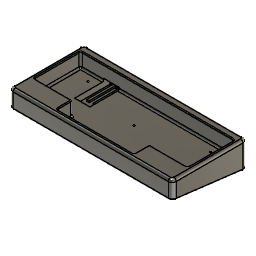
case-file (Autodesk Fusion 360 design; units mm, degrees)
Autodesk Fusion 360 part; units mm, degrees
sketch "Sketch1" plane through (0, 0, 0) normal (0, 0, 1) x (1, 0, 0)
  line L0 (0.9508, 78.7767) -> (191.4508, 78.7767)
  line L1 (0.4508, 79.2767) -> (191.9508, 79.2767)
  line L2 (60.6255, 57.2023) -> (74.6248, 57.2023)
  line L3 (79.6755, 57.2023) -> (93.6748, 57.2023)
  line L4 (0.9508, 89.2767) -> (191.4508, 89.2767)
  line L5 (60.6255, 76.2523) -> (74.6248, 76.2523)
  line L6 (55.5748, 62.253) -> (41.5755, 62.253)
  line L7 (79.6755, 24.1528) -> (79.6755, 38.1522)
  line L8 (60.6255, 24.1528) -> (60.6255, 38.1522)
  line L9 (41.5755, 57.2023) -> (55.5748, 57.2023)
  line L10 (55.5748, 57.2023) -> (55.5748, 43.203)
  line L11 (191.9508, 2.0769) -> (0.4508, 2.0769)
  line L12 (79.6755, 62.253) -> (79.6755, 76.2523)
  line L13 (136.8258, 62.253) -> (136.8258, 76.2523)
  line L14 (117.7738, 76.2523) -> (131.7748, 76.2523)
  line L15 (150.8248, 57.2023) -> (150.8248, 43.203)
  line L16 (131.7748, 24.1528) -> (117.7738, 24.1528)
  line L17 (74.6248, 76.2523) -> (74.6248, 62.253)
  line L18 (131.7748, 43.203) -> (117.7738, 43.203)
  line L19 (188.9248, 43.203) -> (174.9258, 43.203)
  line L20 (79.6755, 43.203) -> (79.6755, 57.2023)
  line L21 (3.4754, 62.253) -> (3.4754, 76.2523)
  line L22 (188.9248, 62.253) -> (174.9258, 62.253)
  line L23 (67.4811, 5.1029) -> (53.4818, 5.1029)
  line L24 (117.7738, 43.203) -> (117.7738, 57.2023)
  line L25 (112.7248, 24.1528) -> (98.7241, 24.1528)
  line L26 (131.7748, 57.2023) -> (131.7748, 43.203)
  line L27 (191.4508, 78.7767) -> (191.4508, 2.5769)
  line L28 (101.1068, 5.1029) -> (101.1068, 19.1023)
  line L29 (155.8758, 24.1528) -> (155.8758, 38.1522)
  line L30 (0.9508, 89.2767) -> (-5.5492, 89.2767)
  line L31 (155.8758, 62.253) -> (155.8758, 76.2523)
  line L32 (144.3188, 5.1029) -> (144.3188, 2.0769)
  line L33 (112.7248, 62.253) -> (98.7241, 62.253)
  line L34 (98.7241, 57.2023) -> (112.7248, 57.2023)
  line L35 (22.5255, 24.1528) -> (22.5255, 38.1522)
  line L36 (41.5755, 62.253) -> (41.5755, 76.2523)
  line L37 (136.8258, 43.203) -> (136.8258, 57.2023)
  line L38 (17.475, 43.203) -> (3.4754, 43.203)
  line L39 (115.1058, 19.1023) -> (115.1058, 5.1029)
  line L40 (188.9248, 57.2023) -> (188.9248, 43.203)
  line L41 (77.2929, 5.1029) -> (77.2929, 19.1023)
  line L42 (48.0818, 5.1029) -> (48.0818, 2.0769)
  line L43 (48.0818, 21.1278) -> (48.0818, 5.1029)
  line L44 (174.9258, 43.203) -> (174.9258, 57.2023)
  line L45 (155.8758, 43.203) -> (155.8758, 57.2023)
  line L46 (74.6248, 38.1522) -> (74.6248, 24.1528)
  line L47 (36.5248, 24.1528) -> (22.5255, 24.1528)
  line L48 (191.9508, 79.2767) -> (191.9508, 2.0769)
  line L49 (150.8248, 76.2523) -> (150.8248, 62.253)
  line L50 (36.5248, 43.203) -> (22.5255, 43.203)
  line L51 (169.8748, 24.1528) -> (155.8758, 24.1528)
  line L52 (143.8188, 5.1029) -> (143.8188, 2.0769)
  line L53 (3.4754, 24.1528) -> (3.4754, 38.1522)
  line L54 (115.1058, 5.1029) -> (101.1068, 5.1029)
  line L55 (138.9188, 5.1029) -> (124.9178, 5.1029)
  line L56 (197.9508, 85.2767) -> (197.9508, -3.9231)
  line L57 (188.9248, 76.2523) -> (188.9248, 62.253)
  line L58 (188.9248, 38.1522) -> (188.9248, 24.1528)
  line L59 (188.9248, 24.1528) -> (174.9258, 24.1528)
  line L60 (112.7248, 76.2523) -> (112.7248, 62.253)
  line L61 (101.1068, 19.1023) -> (115.1058, 19.1023)
  line L62 (169.8748, 43.203) -> (155.8758, 43.203)
  line L63 (48.5818, 21.6278) -> (48.5818, 5.1029)
  line L64 (17.475, 24.1528) -> (3.4754, 24.1528)
  line L65 (77.2929, 19.1023) -> (91.2936, 19.1023)
  line L66 (144.3188, 21.1278) -> (144.3188, 5.1029)
  line L67 (22.5255, 57.2023) -> (36.5248, 57.2023)
  line L68 (174.9258, 24.1528) -> (174.9258, 38.1522)
  line L69 (60.6255, 43.203) -> (60.6255, 57.2023)
  line L70 (174.9258, 57.2023) -> (188.9248, 57.2023)
  line L71 (3.4754, 57.2023) -> (17.475, 57.2023)
  line L72 (79.6755, 76.2523) -> (93.6748, 76.2523)
  line L73 (3.4754, 21.1278) -> (48.0818, 21.1278)
  line L74 (60.6255, 62.253) -> (60.6255, 76.2523)
  line L75 (136.8258, 24.1528) -> (136.8258, 38.1522)
  line L76 (174.9258, 62.253) -> (174.9258, 76.2523)
  line L77 (91.2936, 5.1029) -> (77.2929, 5.1029)
  line L78 (124.9178, 19.1023) -> (138.9188, 19.1023)
  line L79 (93.6748, 38.1522) -> (93.6748, 24.1528)
  line L80 (112.7248, 43.203) -> (98.7241, 43.203)
  line L81 (74.6248, 62.253) -> (60.6255, 62.253)
  line L82 (117.7738, 38.1522) -> (131.7748, 38.1522)
  line L83 (53.4818, 5.1029) -> (53.4818, 19.1023)
  line L84 (138.9188, 19.1023) -> (138.9188, 5.1029)
  line L85 (3.4754, 21.6278) -> (48.5818, 21.6278)
  line L86 (93.6748, 43.203) -> (79.6755, 43.203)
  line L87 (131.7748, 62.253) -> (117.7738, 62.253)
  line L88 (98.7241, 43.203) -> (98.7241, 57.2023)
  line L89 (124.9178, 5.1029) -> (124.9178, 19.1023)
  line L90 (98.7241, 62.253) -> (98.7241, 76.2523)
  line L91 (79.6755, 38.1522) -> (93.6748, 38.1522)
  line L92 (169.8748, 62.253) -> (155.8758, 62.253)
  line L93 (36.5248, 62.253) -> (22.5255, 62.253)
  line L94 (155.8758, 76.2523) -> (169.8748, 76.2523)
  line L95 (3.4754, 76.2523) -> (17.475, 76.2523)
  line L96 (-5.5492, 89.2767) -> (-5.5492, 85.2767)
  line L97 (3.4754, 38.1522) -> (17.475, 38.1522)
  line L98 (112.7248, 38.1522) -> (112.7248, 24.1528)
  line L99 (36.5248, 38.1522) -> (36.5248, 24.1528)
  line L100 (22.5255, 76.2523) -> (36.5248, 76.2523)
  line L101 (112.7248, 57.2023) -> (112.7248, 43.203)
  line L102 (48.5818, 5.1029) -> (48.5818, 2.0769)
  line L103 (98.7241, 76.2523) -> (112.7248, 76.2523)
  line L104 (22.5255, 62.253) -> (22.5255, 76.2523)
  line L105 (22.5255, 38.1522) -> (36.5248, 38.1522)
  line L106 (117.7738, 62.253) -> (117.7738, 76.2523)
  line L107 (188.9248, 21.1278) -> (191.9508, 21.1278)
  line L108 (36.5248, 76.2523) -> (36.5248, 62.253)
  line L109 (53.4818, 19.1023) -> (67.4811, 19.1023)
  line L110 (17.475, 57.2023) -> (17.475, 43.203)
  line L111 (17.475, 38.1522) -> (17.475, 24.1528)
  line L112 (131.7748, 38.1522) -> (131.7748, 24.1528)
  line L113 (98.7241, 24.1528) -> (98.7241, 38.1522)
  line L114 (143.8188, 21.6278) -> (143.8188, 5.1029)
  line L115 (131.7748, 76.2523) -> (131.7748, 62.253)
  line L116 (3.4754, 21.6278) -> (0.4508, 21.6278)
  line L117 (117.7738, 57.2023) -> (131.7748, 57.2023)
  line L118 (41.5755, 24.1528) -> (41.5755, 38.1522)
  line L119 (93.6748, 24.1528) -> (79.6755, 24.1528)
  line L120 (17.475, 62.253) -> (3.4754, 62.253)
  line L121 (17.475, 76.2523) -> (17.475, 62.253)
  line L122 (197.9508, 89.2767) -> (197.9508, 85.2767)
  line L123 (3.4754, 21.1278) -> (0.4508, 21.1278)
  line L124 (98.7241, 38.1522) -> (112.7248, 38.1522)
  line L125 (155.8758, 57.2023) -> (169.8748, 57.2023)
  line L126 (169.8748, 57.2023) -> (169.8748, 43.203)
  line L127 (188.9248, 21.6278) -> (191.9508, 21.6278)
  line L128 (155.8758, 38.1522) -> (169.8748, 38.1522)
  line L129 (174.9258, 38.1522) -> (188.9248, 38.1522)
  line L130 (169.8748, 38.1522) -> (169.8748, 24.1528)
  line L131 (169.8748, 76.2523) -> (169.8748, 62.253)
  line L132 (174.9258, 76.2523) -> (188.9248, 76.2523)
  line L133 (191.4508, 89.2767) -> (197.9508, 89.2767)
  line L134 (150.8248, 38.1522) -> (150.8248, 24.1528)
  line L135 (93.6748, 62.253) -> (79.6755, 62.253)
  line L136 (150.8248, 62.253) -> (136.8258, 62.253)
  line L137 (41.5755, 76.2523) -> (55.5748, 76.2523)
  line L138 (22.5255, 43.203) -> (22.5255, 57.2023)
  line L139 (136.8258, 38.1522) -> (150.8248, 38.1522)
  line L140 (3.4754, 43.203) -> (3.4754, 57.2023)
  line L141 (55.5748, 76.2523) -> (55.5748, 62.253)
  line L142 (136.8258, 57.2023) -> (150.8248, 57.2023)
  line L143 (0.4508, 2.0769) -> (0.4508, 79.2767)
  line L144 (36.5248, 57.2023) -> (36.5248, 43.203)
  line L145 (41.5755, 43.203) -> (41.5755, 57.2023)
  line L146 (150.8248, 24.1528) -> (136.8258, 24.1528)
  line L147 (60.6255, 38.1522) -> (74.6248, 38.1522)
  line L148 (55.5748, 24.1528) -> (41.5755, 24.1528)
  line L149 (188.9248, 21.6278) -> (143.8188, 21.6278)
  line L150 (55.5748, 38.1522) -> (55.5748, 24.1528)
  line L151 (91.2936, 19.1023) -> (91.2936, 5.1029)
  line L152 (74.6248, 57.2023) -> (74.6248, 43.203)
  line L153 (0.9508, 2.5769) -> (0.9508, 78.7767)
  line L154 (117.7738, 24.1528) -> (117.7738, 38.1522)
  line L155 (55.5748, 43.203) -> (41.5755, 43.203)
  line L156 (74.6248, 24.1528) -> (60.6255, 24.1528)
  line L157 (-5.5492, -3.9231) -> (-5.5492, 85.2767)
  line L158 (74.6248, 43.203) -> (60.6255, 43.203)
  line L159 (136.8258, 76.2523) -> (150.8248, 76.2523)
  line L160 (41.5755, 38.1522) -> (55.5748, 38.1522)
  line L161 (93.6748, 57.2023) -> (93.6748, 43.203)
  line L162 (188.9248, 21.1278) -> (144.3188, 21.1278)
  line L163 (93.6748, 76.2523) -> (93.6748, 62.253)
  line L164 (150.8248, 43.203) -> (136.8258, 43.203)
  line L165 (67.4811, 19.1023) -> (67.4811, 5.1029)
  line L166 (191.4508, 2.5769) -> (0.9508, 2.5769)
  line L167 (197.9508, -3.9231) -> (-5.5492, -3.9231)
  line L168 (17.475, 69.2527) -> (22.5255, 69.2527) construction
  line L169 (17.475, 31.1525) -> (22.5255, 31.1525) construction
  line L170 (67.4811, 12.1026) -> (77.2929, 12.1026) construction
  line L171 (93.6748, 50.2027) -> (98.7241, 50.2027) construction
  line L172 (96.2008, 78.7767) -> (96.2008, 2.5769) construction
  circle A0 centre (20.0002, 69.2527) radius 0.75
  circle A1 centre (20.0002, 31.1525) radius 0.75
  circle A2 centre (72.387, 12.1026) radius 0.75
  circle A3 centre (96.1994, 50.2027) radius 0.75
  line L173 (174.9266, 69.2527) -> (169.8761, 69.2527) construction
  circle A4 centre (172.4014, 69.2527) radius 0.75
  line L174 (174.9266, 31.1525) -> (169.8761, 31.1525) construction
  circle A5 centre (172.4014, 31.1525) radius 0.75
  circle A6 centre (120.0146, 12.1026) radius 0.75
  line L175 (124.9205, 12.1026) -> (115.1087, 12.1026) construction
  dimension "d1" = -0.5
  dimension "d3" = -10.5
  dimension "d9" = 0.5
  dimension "d5" = 6.5
  dimension "d6" = 6.5
  dimension "d7" = 6.5
  dimension "d8" = 0.5
  dimension "d10" = 0.5
  dimension "d11" = 0.5
  dimension "d28" = 1.5
  dimension "d29" = 1.5
  dimension "d30" = 1.5
  dimension "d31" = 1.5
  constraint horizontal L30
  constraint vertical L96
  constraint horizontal L133
  constraint vertical L122
  constraint coincident L123.end L143
  constraint perpendicular L123 L143
  constraint perpendicular L43 L73
  constraint perpendicular L75 L149
  constraint perpendicular L114 L149
  constraint coincident L102.end L11
  constraint perpendicular L11 L102
  constraint coincident L42.end L11
  constraint perpendicular L11 L42
  constraint coincident L127.end L48
  constraint perpendicular L48 L127
  constraint coincident L52.end L11
  constraint perpendicular L11 L52
  constraint midpoint L121 L168.start
  constraint midpoint L104 L168.end
  constraint perpendicular L104 L168
  constraint midpoint L111 L169.start
  constraint midpoint L35 L169.end
  constraint midpoint L165 L170.start
  constraint midpoint L41 L170.end
  constraint perpendicular L41 L170
  constraint midpoint L161 L171.start
  constraint midpoint L88 L171.end
  constraint midpoint L0 L172.start
  constraint midpoint L166 L172.end
  constraint perpendicular L166 L172
  constraint midpoint L168 A0.centre
  constraint midpoint L169 A1.centre
  constraint midpoint L170 A2.centre
  constraint midpoint L171 A3.centre
  constraint symmetric L168.start L172 L173.start
  constraint symmetric L168.end L172 L173.end
  constraint symmetric L169.start L172 L174.start
  constraint symmetric L169.end L172 L174.end
  constraint symmetric L170.start L172 L175.start
  constraint symmetric L170.end L172 L175.end
  constraint symmetric L172 A0 A4
  constraint symmetric L172 A1 A5
  constraint symmetric L172 A2 A6
  measures "d5" distance of L153 L157
  measures "d6" distance of L27 L56
  measures "d7" distance of L166 L167
  measures "d8" distance of L116 L123
  measures "d10" distance of L73 L85
  measures "d11" distance of L43 L63
  measures "d28" diameter of A0
  measures "d29" diameter of A1
  measures "d30" diameter of A2
  measures "d31" diameter of A3
extrude "Extrude1" add sketch "Sketch1" along normal blind 10 contours L11 L42 L123 L143 L153 L166 | L42 L43 L73 L123 L153 L166 | L11 L27 L32 L48 L107 L166 | L27 L32 L66 L107 L162 L166 | L4 L30 L56 L96 L122 L133 L157 L167 makes body 1
sketch "Sketch2" plane through (197.9508, 0, 0) normal (1, 0, 0) x (0, 1, 0)
  line L0 (-3.9231, 0) -> (89.2767, 0)
  line L1 (89.2767, 0) -> (89.2767, 10)
  line L2 (89.2767, 10) -> (-3.9231, 10)
  line L3 (-3.9231, 10) -> (-3.9231, 0)
  line L4 (-3.9231, 10) -> (-3.9231, 0)
  line L5 (-3.9231, 0) -> (-3.9231, -12.5)
  line L6 (-3.9231, 0) -> (89.2767, 0)
  line L7 (-3.9231, -12.5) -> (89.2767, -23.9435)
  line L8 (-3.9231, -12.5) -> (89.2767, -12.5) construction
  line L9 (89.2767, 0) -> (89.2767, -23.9435)
  dimension "d18" = 10
  dimension "d19" = 12.5
  dimension "d20" = 7
  constraint coincident L2.end L3.start
  constraint perpendicular L2 L4
  constraint perpendicular L0 L5
  constraint coincident L0.start L3.end
  constraint coincident L0.end L1.start
  constraint horizontal L8
  constraint coincident L7 L9.end
  constraint perpendicular L8 L9
  constraint coincident L8.end L9
  measures "d18" distance of L2.end L0.start
  measures "d19" distance of L0.start L5.end
  measures "d20" angle of L7 L8
extrude "Extrude2" add sketch "Sketch2" against normal blind 210 contours L0 L5 L6 L7 L9 bodies 1
sketch "Sketch3" plane through (0, -3.9231, 0) normal (0, -1, 0) x (1, 0, 0)
  line L0 (197.9508, -12.5) -> (197.9508, 10)
  line L1 (197.9508, 10) -> (-5.5492, 10)
  line L2 (-5.5492, 10) -> (-5.5492, 0)
  line L3 (-5.5492, 0) -> (-12.0492, 0)
  line L4 (-12.0492, 0) -> (-12.0492, -12.5)
  line L5 (-12.0492, -12.5) -> (197.9508, -12.5)
  line L6 (-5.5492, 10) -> (-27, 10)
  line L7 (-27, 10) -> (-27, -25)
  line L8 (-27, -25) -> (-5.5492, -25)
  line L9 (-5.5492, -25) -> (-5.5492, 10)
  constraint horizontal L6
  constraint vertical L7
  constraint horizontal L8
  constraint vertical L9
  constraint coincident L1.end L2.start
extrude "Extrude3" cut sketch "Sketch3" against normal through all contours L2 L3 L4 L5 L6 L7 L8 L9 | L3 L4 L5 L9 bodies 1
extrude "Extrude4" cut 1 faces at (112.2401, 59.8938, 0) along direction (0, 0, -1) blind 8 on bodies 1 bodies 1
extrude "Extrude5" add sketch "Sketch1" along normal blind 3 separate body contours L0 L27 L52 L63 L85 L102 L114 L116 L127 L149 L153 L166 | A0 | A1 | A2 | A3 | A4 | A5 | A6 makes body 2
extrude "Extrude6" cut sketch "Sketch1" against normal through all contours A0 | A1 | A2 | A3 | A4 | A5 | A6 bodies 1
sketch "Sketch4" plane through (0, 0, -8) normal (0, 0, 1) x (-1, 0, 0)
  circle A0 centre (-120.0146, -12.1026) radius 0.75
  circle A1 centre (-20.0002, -69.2527) radius 0.75
  circle A2 centre (-96.1994, -50.2027) radius 0.75
  circle A3 centre (-172.4014, -69.2527) radius 0.75
  circle A4 centre (-20.0002, -31.1525) radius 0.75
  circle A5 centre (-72.387, -12.1026) radius 0.75
  circle A6 centre (-172.4014, -31.1525) radius 0.75
  line L0 (-48.0818, -21.1278) -> (-48.0818, -2.0769)
  line L1 (-48.0818, -2.0769) -> (-144.3188, -2.0769)
  line L2 (-144.3188, -2.0769) -> (-144.3188, -21.1278)
  line L3 (-144.3188, -21.1278) -> (-191.9508, -21.1278)
  line L4 (-191.9508, -21.1278) -> (-191.9508, -79.2767)
  line L5 (-191.9508, -79.2767) -> (-0.4508, -79.2767)
  line L6 (-0.4508, -79.2767) -> (-0.4508, -21.1278)
  line L7 (-0.4508, -21.1278) -> (-48.0818, -21.1278)
  circle A7 centre (-20.0002, -69.2527) radius 3.5
  circle A8 centre (-20.0002, -31.1525) radius 3.5
  circle A9 centre (-72.387, -12.1026) radius 3.5
  circle A10 centre (-96.1994, -50.2027) radius 3.5
  circle A11 centre (-120.0146, -12.1026) radius 3.5
  circle A12 centre (-172.4014, -31.1525) radius 3.5
  circle A13 centre (-172.4014, -69.2527) radius 3.5
  circle A14 centre (-20.0002, -69.2527) radius 1.25
  circle A15 centre (-20.0002, -31.1525) radius 1.25
  circle A16 centre (-72.387, -12.1026) radius 1.25
  circle A17 centre (-120.0146, -12.1026) radius 1.25
  circle A18 centre (-96.1994, -50.2027) radius 1.25
  circle A19 centre (-172.4014, -31.1525) radius 1.25
  circle A20 centre (-172.4014, -69.2527) radius 1.25
  dimension "d33" = 7
  dimension "d34" = 7
  dimension "d35" = 7
  dimension "d36" = 7
  dimension "d37" = 7
  dimension "d38" = 7
  dimension "d39" = 7
  dimension "d40" = 2.5
  dimension "d41" = 2.5
  dimension "d42" = 2.5
  dimension "d43" = 2.5
  dimension "d44" = 2.5
  dimension "d45" = 2.5
  dimension "d46" = 2.5
  constraint concentric A1 A7
  constraint concentric A4 A8
  constraint concentric A5 A9
  constraint concentric A2 A10
  constraint concentric A0 A11
  constraint concentric A6 A12
  constraint concentric A3 A13
  constraint concentric A1 A14
  constraint concentric A8 A15
  constraint concentric A9 A16
  constraint concentric A11 A17
  constraint concentric A10 A18
  constraint concentric A12 A19
  constraint concentric A13 A20
  measures "d33" diameter of A7
  measures "d34" diameter of A8
  measures "d35" diameter of A9
  measures "d36" diameter of A10
  measures "d37" diameter of A11
  measures "d38" diameter of A12
  measures "d39" diameter of A13
  measures "d40" diameter of A14
  measures "d41" diameter of A15
  measures "d42" diameter of A16
  measures "d43" diameter of A17
  measures "d44" diameter of A18
  measures "d45" diameter of A19
  measures "d46" diameter of A20
extrude "Extrude7" cut sketch "Sketch4" against normal through all contours A7 | A8 | A9 | A10 | A11 | A12 | A13 | A14 | A15 | A16 | A17 | A18 | A19 | A20 bodies 1
extrude "Extrude8" add sketch "Sketch4" against normal blind 2 contours A7 | A8 | A9 | A10 | A11 | A12 | A13 bodies 1
sketch "Sketch5" plane through (0, 0, -8) normal (0, 0, 1) x (-1, 0, 0)
  circle A0 centre (-20.0002, -69.2527) radius 1.25
  circle A1 centre (-120.0146, -12.1026) radius 1.25
  circle A2 centre (-172.4014, -31.1525) radius 1.25
  circle A3 centre (-20.0002, -31.1525) radius 1.25
  circle A4 centre (-96.1994, -50.2027) radius 1.25
  circle A5 centre (-172.4014, -69.2527) radius 1.25
  circle A6 centre (-72.387, -12.1026) radius 1.25
  line L0 (-48.0818, -21.1278) -> (-48.0818, -2.0769)
  line L1 (-48.0818, -2.0769) -> (-144.3188, -2.0769)
  line L2 (-144.3188, -2.0769) -> (-144.3188, -21.1278)
  line L3 (-144.3188, -21.1278) -> (-191.9508, -21.1278)
  line L4 (-191.9508, -21.1278) -> (-191.9508, -79.2767)
  line L5 (-191.9508, -79.2767) -> (-0.4508, -79.2767)
  line L6 (-0.4508, -79.2767) -> (-0.4508, -21.1278)
  line L7 (-0.4508, -21.1278) -> (-48.0818, -21.1278)
  line L8 (-0.4508, -50.2023) -> (-29.5508, -50.2023) construction
  line L9 (-29.5508, -50.2023) -> (-29.5508, -79.2767) construction
  line L10 (-29.5508, -79.2767) -> (-48.5508, -79.2767)
  line L11 (-29.5508, -79.2767) -> (-29.5508, -50.2023)
  line L12 (-29.5508, -50.2023) -> (-48.5508, -50.2023)
  line L13 (-48.5508, -50.2023) -> (-48.5508, -79.2767)
  dimension "d50" = 29.1
  dimension "d51" = 19
  dimension "d52" = 19
  constraint midpoint L6 L8.start
  constraint perpendicular L6 L8
  constraint coincident L5 L9.end
  constraint perpendicular L5 L9
  constraint perpendicular L9 L10
  constraint perpendicular L11 L12
  measures "d50" distance of L8.start L8.end
  measures "d51" distance of L9.end L10.end
  measures "d52" distance of L8.end L12.end
extrude "Extrude9" cut sketch "Sketch5" against normal blind 7 contours L5 L10 L11 L12 L13 bodies 1
sketch "Sketch6" plane through (0, 79.2767, 0) normal (0, -1, 0) x (1, 0, 0)
  line L0 (191.9508, -8) -> (191.9508, 10)
  line L1 (191.9508, 10) -> (0.4508, 10)
  line L2 (0.4508, 10) -> (0.4508, -8)
  line L3 (0.4508, -8) -> (29.5508, -8)
  line L4 (29.5508, -8) -> (29.5508, -15)
  line L5 (29.5508, -15) -> (48.5508, -15)
  line L6 (48.5508, -15) -> (48.5508, -8)
  line L7 (48.5508, -8) -> (191.9508, -8)
  line L8 (29.5508, -8) -> (29.5508, -5)
  line L9 (48.5508, -8) -> (48.5508, -5)
  line L10 (29.5508, -5) -> (48.5508, -5)
  dimension "d63" = 3
  dimension "d64" = 3
  constraint coincident L3.end L4.start
  constraint perpendicular L3 L8
  constraint coincident L6.end L7.start
  constraint perpendicular L7 L9
  measures "d63" distance of L3.end L8.end
  measures "d64" distance of L6.end L9.end
extrude "Extrude13" cut sketch "Sketch6" against normal blind 7.5 contours L4 L5 L6 L8 L9 L10 bodies 1
extrude "Extrude14" cut 1 faces at (42.2175, 86.7767, -11.6667) along direction (0, -1, 0) blind 44 on bodies 1 bodies 1
sketch "Sketch7" plane through (0, 0, -15) normal (0, 0, 1) x (-1, 0, 0)
  line L0 (-29.5508, -86.7767) -> (-29.5508, -42.7767)
  line L1 (-29.5508, -42.7767) -> (-48.5508, -42.7767)
  line L2 (-48.5508, -42.7767) -> (-48.5508, -86.7767)
  line L3 (-48.5508, -86.7767) -> (-29.5508, -86.7767)
  line L4 (-29.5508, -86.7767) -> (-33.5508, -86.7767) construction
  line L5 (-33.5508, -86.7767) -> (-33.5508, -53.7767)
  line L6 (-33.5508, -53.7767) -> (-36.5508, -53.7767)
  line L7 (-36.5508, -53.7767) -> (-36.5508, -86.7767)
  line L8 (-48.5508, -86.7767) -> (-44.5508, -86.7767) construction
  line L9 (-44.5508, -86.7767) -> (-44.5508, -53.7767)
  line L10 (-44.5508, -53.7767) -> (-41.5508, -53.7767)
  line L11 (-41.5508, -53.7767) -> (-41.5508, -86.7767)
  line L12 (-39.0508, -42.7767) -> (-39.0508, -47.7767) construction
  circle A0 centre (-39.0508, -47.7767) radius 1.25
  circle A1 centre (-39.0508, -47.7767) radius 3.5
  dimension "d69" = 4
  dimension "d70" = 33
  dimension "d71" = 3
  dimension "d72" = 4
  dimension "d73" = 33
  dimension "d74" = 3
  dimension "d75" = 5
  dimension "d76" = 2.5
  dimension "d77" = 7
  constraint coincident L0.start L3.end
  constraint perpendicular L0 L4
  constraint perpendicular L4 L5
  constraint perpendicular L5 L6
  constraint coincident L3 L7.end
  constraint perpendicular L3 L7
  constraint coincident L2.end L3.start
  constraint perpendicular L2 L8
  constraint perpendicular L8 L9
  constraint perpendicular L9 L10
  constraint coincident L3 L11.end
  constraint perpendicular L3 L11
  constraint midpoint L1 L12.start
  constraint perpendicular L1 L12
  constraint coincident L12.end A0.centre
  constraint concentric A0 A1
  measures "d69" distance of L0.start L4.end
  measures "d70" distance of L4.end L5.end
  measures "d71" distance of L5.end L6.end
  measures "d72" distance of L2.end L8.end
  measures "d73" distance of L8.end L9.end
  measures "d74" distance of L9.end L10.end
  measures "d75" distance of L12.start L12.end
  measures "d76" diameter of A0
  measures "d77" diameter of A1
extrude "Extrude15" add sketch "Sketch7" along normal blind 2 contours L3 L5 L6 L7 | L3 L9 L10 L11 bodies 1
extrude "Extrude16" cut sketch "Sketch7" against normal through all contours A0 | A1 bodies 1
extrude "Extrude18" add sketch "Sketch7" against normal blind 1.5 contours A1 bodies 1
sketch "Sketch8" plane through (0, 86.7767, 0) normal (0, -1, 0) x (1, 0, 0)
  line L0 (41.5508, -15) -> (41.5508, -13)
  line L1 (41.5508, -13) -> (44.5508, -13)
  line L2 (44.5508, -13) -> (44.5508, -15)
  line L3 (44.5508, -15) -> (48.5508, -15)
  line L4 (48.5508, -15) -> (48.5508, -5)
  line L5 (48.5508, -5) -> (29.5508, -5)
  line L6 (29.5508, -5) -> (29.5508, -15)
  line L7 (29.5508, -15) -> (33.5508, -15)
  line L8 (33.5508, -15) -> (33.5508, -13)
  line L9 (33.5508, -13) -> (36.5508, -13)
  line L10 (36.5508, -13) -> (36.5508, -15)
  line L11 (36.5508, -15) -> (41.5508, -15)
  line L12 (39.0508, -15) -> (39.0508, -11.75) construction
  line L13 (39.0508, -11.75) -> (42.7508, -11.75)
  line L14 (39.0508, -11.75) -> (35.3508, -11.75)
  line L15 (35.3508, -11.75) -> (35.3508, -9)
  line L16 (42.7508, -11.75) -> (42.7508, -9)
  line L17 (35.3508, -9) -> (35.5, -9)
  line L18 (35.5, -9) -> (42.7508, -9)
  dimension "d85" = 3.25
  dimension "d86" = 3.7
  dimension "d87" = 3.7
  dimension "d88" = 2.75
  dimension "d89" = 2.75
  constraint midpoint L11 L12.start
  constraint perpendicular L11 L12
  constraint perpendicular L12 L13
  constraint perpendicular L12 L14
  constraint perpendicular L14 L15
  constraint perpendicular L13 L16
  constraint perpendicular L15 L17
  measures "d85" distance of L12.start L12.end
  measures "d86" distance of L12.end L13.end
  measures "d87" distance of L12.end L14.end
  measures "d88" distance of L14.end L15.end
  measures "d89" distance of L13.end L16.end
extrude "Extrude19" cut sketch "Sketch8" against normal through all contours L13 L14 L15 L16 L17 L18 bodies 1
fillet "Fillet1" radius 5 4 edges at (197.9508, -3.9231, -1.25) (197.9508, 89.2767, -6.9717) (-5.5492, 89.2767, -6.9717) (-5.5492, -3.9231, -1.25) on bodies 1
fillet "Fillet1" radius 2 8 edges at (0.4508, 79.2767, 1) (191.9508, 79.2767, 1) (191.9508, 21.1278, 1) (0.4508, 21.1278, 1) (48.0818, 2.0769, 1) (144.3188, 2.0769, 1) (144.3188, 21.1278, 1) (48.0818, 21.1278, 1) on bodies 1
fillet "Fillet1" radius 2 4 edges at (96.2008, 89.2767, -23.9435) (-5.5492, 42.6768, -18.2217) (96.2008, -3.9231, -12.5) (197.9508, 42.6768, -18.2217) on bodies 1
fillet "Fillet1" radius 3 4 edges at (96.2008, -3.9231, 10) (197.9508, 42.6768, 10) (96.2008, 89.2767, 10) (-5.5492, 42.6768, 10) on bodies 1
fillet "Fillet1" radius 1 8 edges at (0.4508, 50.2023, 10) (96.2008, 79.2767, 10) (24.2663, 21.1278, 10) (48.0818, 11.6024, 10) (96.2003, 2.0769, 10) (191.9508, 50.2023, 10) (168.1348, 21.1278, 10) (144.3188, 11.6024, 10) on bodies 1
fillet "Fillet1" radius 2 9 edges at (15.0008, 79.2767, -8) (120.2508, 79.2767, -8) (191.9508, 50.2023, -8) (168.1348, 21.1278, -8) (144.3188, 11.6024, -8) (96.2003, 2.0769, -8) (48.0818, 11.6024, -8) (24.2663, 21.1278, -8) (0.4508, 50.2023, -8) on bodies 1
fillet "Fillet1" radius 0.5 12 edges at (39.0508, 89.2767, -11.75) (42.7508, 89.2767, -10.375) (39.0508, 89.2767, -9) (35.3508, 89.2767, -10.375) (42.7508, 88.0267, -11.75) (35.3508, 88.0267, -11.75) (35.3508, 88.0267, -9) (42.7508, 88.0267, -9) (39.0508, 86.7767, -11.75) (35.3508, 86.7767, -10.375) (42.7508, 86.7767, -10.375) (39.0508, 86.7767, -9) on bodies 1
fillet "Fillet1" radius 1 4 edges at (31.5508, 86.7767, -15) (39.0508, 86.7767, -15) (46.5508, 86.7767, -15) (39.0508, 86.7767, -5) on bodies 1
hidden bodies 2
